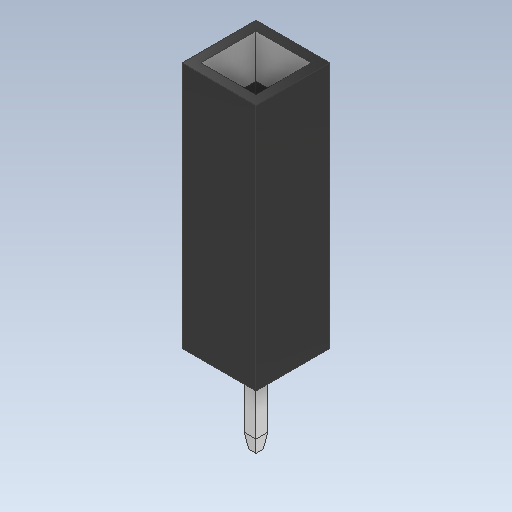
# Autodesk Inventor part: FemaleHederPin
Saved by Autodesk Inventor 2020 (Build 240168000, 168)
## iProperties
Created: 2020-01-02
Part Number: FemaleHederPin
Material: Generic
Document SubType Name: Modeling
Designer: ermoz
Density: 1 g/cm^3
Appearance: Default
Mass: 0.0534802 g
Surface Area: 1.12055 cm^2
Volume: 0.0534802 cm^3
Author: ermoz
Autodesk Inventor part; units mm, degrees
ref_plane "YZ Plane" through (0, 0, 0) normal (1, 0, 0) x (0, 1, 0)
ref_plane "XZ Plane" through (0, 0, 0) normal (0, 1, 0) x (-1, 0, 0)
ref_plane "XY Plane" through (0, 0, 0) normal (0, 0, 1) x (1, 0, 0)
sketch "Sketch1" plane through (0, 0, 0) normal (0, 1, 0) x (-1, 0, 0)
  line L0 (-1.27, 1.27) -> (1.27, 1.27)
  line L1 (1.27, 1.27) -> (1.27, -1.27)
  line L2 (1.27, -1.27) -> (-1.27, -1.27)
  line L3 (-1.27, -1.27) -> (-1.27, 1.27)
  line L4 (-1.27, 1.27) -> (1.27, -1.27) construction
  line L5 (1.27, 1.27) -> (-1.27, -1.27) construction
  point P0 (0, 0)
  dimension "d0" = 2.54
  dimension "d1" = 2.54
  constraints: 12 end point, 2 midpoint, 2 parallel, 1 horizontal, 1 perpendicular
  measures "d0" distance of L1.end L2.end
  measures "d1" distance of L0.end L1.end
extrude "Extrusion1" add sketch "Sketch1" along normal blind 8.5
sketch "Sketch2" plane through (0, 8.5, 0) normal (0, 1, 0) x (1, 0, 0)
  line L0 (0.2, -0.2) -> (-0.2, -0.2)
  line L1 (-0.2, -0.2) -> (-0.2, 0.2)
  line L2 (-0.2, 0.2) -> (0.2, 0.2)
  line L3 (0.2, 0.2) -> (0.2, -0.2)
  line L4 (0.2, -0.2) -> (-0.2, 0.2) construction
  line L5 (-0.2, -0.2) -> (0.2, 0.2) construction
  point P0 (0, 0)
  dimension "d4" = 0.4
  dimension "d5" = 0.4
  constraints: 12 end point, 2 midpoint, 2 parallel, 1 horizontal, 1 perpendicular
  measures "d4" distance of L1.end L2.end
  measures "d5" distance of L0.end L1.end
extrude "Extrusion2" cut sketch "Sketch2" against normal blind 5
chamfer "Chamfer1" distance 0.75 angle 45 4 edges at (0, 8.5, 0.2) (-0.2, 8.5, 0) (0, 8.5, -0.2) (0.2, 8.5, 0)
sketch "Sketch3" plane through (0, 0, 0) normal (0, -1, 0) x (1, 0, 0)
  line L0 (-0.2, 0.2) -> (0.2, 0.2)
  line L1 (0.2, 0.2) -> (0.2, -0.2)
  line L2 (0.2, -0.2) -> (-0.2, -0.2)
  line L3 (-0.2, -0.2) -> (-0.2, 0.2)
  line L4 (-0.2, 0.2) -> (0.2, -0.2) construction
  line L5 (0.2, 0.2) -> (-0.2, -0.2) construction
  point P0 (0, 0)
  dimension "d11" = 0.4
  dimension "d12" = 0.4
  constraints: 12 end point, 2 midpoint, 2 parallel, 1 horizontal, 1 perpendicular
  measures "d11" distance of L1.end L2.end
  measures "d12" distance of L0.end L1.end
extrude "Extrusion3" add sketch "Sketch3" along normal blind 3
chamfer "Chamfer2" distance 0.074 distance2 0.5 1 edges at (-0.2, -3, 0) measured on face at (-0.0667, -3, 0.0667)
chamfer "Chamfer3" distance 0.074 distance2 0.5 1 edges at (0.2, -3, 0) measured on face at (-0.0173, -3, 0.0667)
chamfer "Chamfer4" distance 0.074 distance2 0.5 1 edges at (0, -3, 0.2) measured on face at (-0.042, -3, 0.0667)
chamfer "Chamfer5" distance 0.074 distance2 0.5 1 edges at (0, -3, -0.2) measured on face at (0.042, -3, -0.0913)
body "Solid1"
